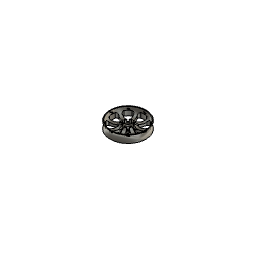
Buffer_Wheel (Autodesk Fusion 360 design; units mm, degrees)
Autodesk Fusion 360 part; units mm, degrees
sketch "Main Wheel Body" plane through (0, 0, 0) normal (0, 0, 1) x (1, 0, 0)
  circle A0 centre (0, 0) radius 44.25
  circle A1 centre (0, 0) radius 11.5
  circle A2 centre (0, 0) radius 39.25
  line L0 (0, 39.25) -> (0, -39.25) construction
  line L1 (0, 11.5) -> (-12.0554, 37.3528)
  line L2 (0, 11.5) -> (12.0554, 37.3528)
  line L3 (0, 37.3528) -> (12.0554, 37.3528) construction
  line L4 (-12.0554, 37.3528) -> (0, 37.3528) construction
  line L5 (-8.1317, 8.1317) -> (-17.888, 34.9368)
  line L6 (-8.1317, 8.1317) -> (-34.9368, 17.888)
  line L7 (-11.5, 0) -> (-37.3528, 12.0554)
  line L8 (-11.5, 0) -> (-37.3528, -12.0554)
  line L9 (-8.1317, -8.1317) -> (-34.9368, -17.888)
  line L10 (-8.1317, -8.1317) -> (-17.888, -34.9368)
  line L11 (0, -11.5) -> (-12.0554, -37.3528)
  line L12 (0, -11.5) -> (12.0554, -37.3528)
  line L13 (8.1317, -8.1317) -> (17.888, -34.9368)
  line L14 (8.1317, -8.1317) -> (34.9368, -17.888)
  line L15 (11.5, 0) -> (37.3528, -12.0554)
  line L16 (11.5, 0) -> (37.3528, 12.0554)
  line L17 (8.1317, 8.1317) -> (34.9368, 17.888)
  line L18 (8.1317, 8.1317) -> (17.888, 34.9368)
  circle A3 centre (0, 0) radius 6.5
  circle A4 centre (0, 0) radius 11
  dimension "d6" = 88.5
  dimension "d7" = 23
  dimension "d8" = 78.5
  dimension "d9" = 50
  dimension "d11" = 360
  dimension "d12" = 13
  dimension "d13" = 22
  constraint coincident A0.centre A1.centre
  constraint coincident A2 L0.start
  constraint coincident A2 L0.end
  constraint vertical L0
  constraint coincident A0.centre L0
  constraint coincident A1 L1.start
  constraint coincident L0 L1.start
  constraint coincident A2 L1.end
  constraint coincident A2 L2.end
  constraint coincident L0 L3.start
  constraint horizontal L3
  constraint horizontal L4
  constraint concentric A1 A3
  measures "d6" diameter of A0
  measures "d7" diameter of A1
  measures "d8" diameter of A2
  measures "d9" angle of L1 L2
  measures "d12" diameter of A3
  measures "d13" diameter of A4
extrude "Extrude1" add sketch "Main Wheel Body" along normal blind 17.95 contours A0 | A1 | A1 A2 L14 L15 | A1 A2 L16 L17 | A1 A2 L2 L18 | A1 A2 L12 L13 | A1 A2 L1 L5 | A1 A2 L10 L11 | A1 A2 L6 L7 | A1 A2 L8 L9
extrude "Extrude2" add sketch "Main Wheel Body" along normal blind 4.725 contours A4
fillet "Fillet1" radius 2 8 edges at (11.5, 0, 8.975) (8.1317, 8.1317, 8.975) (0, 11.5, 8.975) (-8.1317, 8.1317, 8.975) (-11.5, 0, 8.975) (-8.1317, -8.1317, 8.975) (0, -11.5, 8.975) (8.1317, -8.1317, 8.975)
fillet "Fillet1" radius 4 16 edges at (37.3528, 12.0554, 8.975) (34.9368, 17.888, 8.975) (37.3528, -12.0554, 8.975) (17.888, 34.9368, 8.975) (12.0554, 37.3528, 8.975) (-12.0554, 37.3528, 8.975) (-17.888, 34.9368, 8.975) (-34.9368, 17.888, 8.975) (-37.3528, 12.0554, 8.975) (-37.3528, -12.0554, 8.975) (-34.9368, -17.888, 8.975) (-17.888, -34.9368, 8.975) (-12.0554, -37.3528, 8.975) (12.0554, -37.3528, 8.975) (17.888, -34.9368, 8.975) (34.9368, -17.888, 8.975)
sketch "Exterior Scoop" plane through (0, 0, 0) normal (0, 1, 0) x (1, 0, 0)
  line L0 (-44.25, 0) -> (44.25, 0) construction
  line L1 (-44.25, -17.95) -> (44.25, -17.95) construction
  line L2 (0, 0) -> (0, -17.95) construction
  line L3 (0, -8.975) -> (41, -8.975) construction
  arc A0 (44.25, 0) -> (44.25, -17.95) centre (55.0174, -8.975) ccw
  line L4 (44.25, -17.95) -> (44.25, 0)
  dimension "d22" = 41
  constraint coincident L2.start origin
  constraint midpoint L1 L2.end
  constraint midpoint L2 L3.start
  constraint perpendicular L2 L3
  constraint coincident L3.end A0
  constraint coincident L1.end A0.end
  constraint coincident L0.end A0.start
  measures "d22" distance of L3.start L3.end
revolve "Revolve1" cut sketch "Exterior Scoop" angle 360 about axis through (0, 0, 0) along (0, 0, 1)
sketch "Internal Scoop" plane through (0, 0, 0) normal (0, 1, 0) x (1, 0, 0)
  line L0 (32.9757, 0) -> (32.9757, -17.95) construction
  line L1 (32.9757, -17.95) -> (15.3872, -17.95) construction
  line L2 (15.3872, -17.95) -> (15.3872, 0) construction
  line L3 (15.3872, 0) -> (32.9757, 0) construction
  line L4 (38.5999, 0) -> (32.9757, 0) construction
  line L5 (38.5999, 0) -> (38.5999, -17.95) construction
  line L6 (32.9757, -17.95) -> (38.5999, -17.95) construction
  line L7 (32.9757, -17.95) -> (32.9757, 0) construction
  line L8 (38.5999, 0) -> (38.5999, -17.95) construction
  line L9 (39.25, -17.95) -> (38.5999, -17.95) construction
  line L10 (38.5999, -17.95) -> (38.5999, 0) construction
  line L11 (39.25, 0) -> (38.5999, 0) construction
  line L12 (32.9757, -17.95) -> (32.9757, 0) construction
  line L13 (32.9757, 0) -> (15.3872, 0) construction
  line L14 (15.3872, 0) -> (15.3872, -17.95) construction
  line L15 (15.3872, -17.95) -> (32.9757, -17.95) construction
  line L16 (38.5999, 0) -> (32.9757, 0) construction
  line L17 (32.9757, 0) -> (32.9757, -17.95) construction
  line L18 (32.9757, -17.95) -> (38.5999, -17.95) construction
  line L19 (38.5999, -17.95) -> (38.5999, 0) construction
  line L20 (15.3872, 0) -> (14.2324, 0) construction
  line L21 (15.3872, 0) -> (15.3872, -17.95) construction
  line L22 (14.2324, -17.95) -> (15.3872, -17.95) construction
  line L23 (15.3872, -17.95) -> (15.3872, 0) construction
  line L24 (-44.25, -17.95) -> (44.25, -17.95) construction
  line L25 (-44.25, 0) -> (44.25, 0) construction
  circle A0 centre (26.3186, -21.9182) radius 16.4182
  line L26 (42.25, -17.95) -> (42.25, 0) construction
  line L27 (10.3872, -17.95) -> (10.3872, 0) construction
  line L28 (42.25, -5.5) -> (10.3872, -5.5) construction
  line L29 (26.3186, -5.5) -> (26.3186, 0) construction
  line L30 (0, 0) -> (0, -17.95) construction
  dimension "d24" = 2
  dimension "d26" = 5.5
  dimension "d48" = 5
  constraint coincident L24 L26.start
  constraint coincident L25 L26.end
  constraint perpendicular L25 L26
  constraint coincident A0 L26.start
  constraint coincident L26 L28.start
  constraint coincident L27 L28.end
  constraint perpendicular L27 L28
  constraint midpoint L28 L29.start
  constraint coincident L3 L29.end
  constraint perpendicular L13 L29
  constraint coincident A0 L29.start
  constraint coincident L30.start origin
  constraint midpoint L24 L30.end
  constraint coincident A0 L27.start
  constraint vertical L27
  constraint coincident L24 L27.start
  constraint coincident L25 L27.end
  measures "d24" distance of L24.end L26
  measures "d26" distance of L29.start L29.end
  measures "d48" distance of L14 L27
revolve "Revolve2" cut sketch "Internal Scoop" angle 360 about axis through (0, 0, 0) along (0, 0, 1)
sketch "Inner Splines" plane through (0, 0, 17.95) normal (0, 0, 1) x (-1, 0, 0)
  circle A0 centre (0, 0) radius 22.5
  line L0 (0, 0) -> (-4.0909, -22.125)
  line L1 (0, 0) -> (4.0909, -22.125)
  line L2 (4.0909, -22.125) -> (0, -22.125) construction
  line L3 (0, 0) -> (0, -22.5) construction
  line L4 (0, -22.125) -> (-4.0909, -22.125) construction
  line L5 (0, 0) -> (18.5374, -12.752)
  line L6 (0, 0) -> (12.752, -18.5374)
  line L7 (0, 0) -> (22.125, 4.0909)
  line L8 (0, 0) -> (22.125, -4.0909)
  line L9 (0, 0) -> (12.752, 18.5374)
  line L10 (0, 0) -> (18.5374, 12.752)
  line L11 (0, 0) -> (-4.0909, 22.125)
  line L12 (0, 0) -> (4.0909, 22.125)
  line L13 (0, 0) -> (-18.5374, 12.752)
  line L14 (0, 0) -> (-12.752, 18.5374)
  line L15 (0, 0) -> (-22.125, -4.0909)
  line L16 (0, 0) -> (-22.125, 4.0909)
  line L17 (0, 0) -> (-12.752, -18.5374)
  line L18 (0, 0) -> (-18.5374, -12.752)
  circle A1 centre (0, 0) radius 42.25
  circle A2 centre (0, 0) radius 44.25
  circle A3 centre (0, 0) radius 11
  point P0 (2, -10.8167)
  point P1 (-2, -10.8167)
  dimension "d28" = 45
  dimension "d30" = 4
  dimension "d32" = 360
  constraint coincident A0.centre L0.start
  constraint coincident A0 L0.end
  constraint coincident A0 L1.end
  constraint coincident A0 L3.end
  constraint vertical L3
  constraint coincident L3 L2.end
  constraint perpendicular L3 L4
  constraint perpendicular L2 L3
  constraint coincident L1 P0
  constraint coincident L0 P1
  constraint coincident P0 A3
  constraint coincident P1 A3
  measures "d28" diameter of A0
  measures "d30" distance of P0 P1
extrude "Extrude3" cut sketch "Inner Splines" along normal up to surface (12.725 mm away) from surface at -12.725 contours A0 L7 L8 A3 | A0 L9 L10 A3 | L7 L8 A3 | A0 L5 L6 A3 | L9 L10 A3 | L0 L1 A3 | L5 L6 A3 | L11 L12 A3 | L13 L14 A3 | L15 L16 A3 | L17 L18 A3 | A0 L11 L12 A3 | A0 L0 L1 A3 | A0 L13 L14 A3 | A0 L15 L16 A3 | A0 L17 L18 A3
sketch "Center Height Cutoff" plane through (0, 0, 0) normal (0, 0, 1) x (1, 0, 0)
  circle A0 centre (0, 0) radius 22.5
  dimension "d44" = 45
  constraint coincident A0.centre origin
  measures "d44" diameter of A0
extrude "Extrude5" cut sketch "Center Height Cutoff" along normal up to surface (6.075 mm away) from surface at 11.875
ref_plane "WorkPlane1" through (-24.4264, 6.0277, 8.975) normal (-0.422618, -0.906308, 0) x (0.906308, -0.422618, 0)
sketch "Filament Loading Holes" plane through (-2.054, -4.4048, 0) normal (-0.422618, -0.906308, 0) x (0.906308, -0.422618, 0)
  line L0 (44.25, 17.95) -> (-44.25, 17.95) construction
  line L1 (44.25, 0) -> (-44.25, 0) construction
  spline S0 degree 3 poles (-34.1183, 7.6623) (-34.1618, 7.6869) (-34.2052, 7.7118) (-34.3768, 7.8114) (-34.5038, 7.8879) (-34.7611, 8.0488) (-34.8912, 8.1334) (-35.2079, 8.3473) (-35.3915, 8.4786) (-35.965, 8.9119) (-36.3296, 9.2252) (-37.0606, 9.9351) (-37.4074, 10.3389) (-37.8929, 11.0303) (-38.041, 11.3141) (-38.1207, 11.6036) (-38.1258, 11.6785) (-38.0894, 11.777) (-38.0506, 11.8021) (-37.9899, 11.8021) knots 0.31518 0.31518 0.31518 0.31518 0.330141 0.330141 0.374564 0.374564 0.421467 0.421467 0.490968 0.490968 0.646609 0.646609 0.84456 0.84456 1.024108 1.024108 1.108559 1.108559 1.18857 1.18857 1.18857 1.18857 construction
  spline S1 degree 3 poles (-18.7598, 7.0386) (-18.971, 6.9433) (-19.181, 6.8535) (-20.3556, 6.3774) (-21.4495, 6.0412) (-23.683, 5.6024) (-24.8226, 5.5) (-26.898, 5.5) (-28.0254, 5.6002) (-30.2338, 6.035) (-31.3148, 6.3697) (-32.8752, 7.0126) (-33.5024, 7.314) (-34.1183, 7.6623) knots 6.716053 6.716053 6.716053 6.716053 6.783241 6.783241 7.096258 7.096258 7.409274 7.409274 7.718882 7.718882 8.02849 8.02849 8.225182 8.225182 8.225182 8.225182 construction
  line L2 (-37.25, 0) -> (-37.25, 17.95) construction
  circle A0 centre (-37.25, 13.95) radius 1
  dimension "d37" = 7
  dimension "d38" = 2
  dimension "d39" = 4
  constraint coincident L1 L2.start
  constraint coincident L0 L2.end
  constraint perpendicular L0 L2
  constraint coincident L2 A0.centre
  measures "d37" distance of L0.end L2
  measures "d38" diameter of A0
  measures "d39" distance of L2.end A0.centre
extrude "Extrude4" cut sketch "Filament Loading Holes" along normal up to surface end surface at (-43.7914, 2.1855, 17.4418)
pattern_circular "C-Pattern1" count 8 over 360 about axis through (0, 0, -205.75) along (0, 0, 1) of "Extrude4"
equation "d22 = ( 82 / 2 ) * 1 mm"
